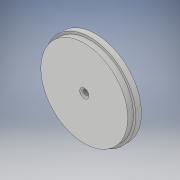
# Autodesk Inventor part: Cap
Saved by Autodesk Inventor 2019 (Build 230136000, 136)
## iProperties
Created: 2021-01-17
Part Number: Cap
Material: Типовые
Document SubType Name: Modeling
Designer: Dazer
Density: 1 g/cm^3
Appearance: По умолчанию
Author: Dazer
## iProperties of the stored document Cap_3DПЕЧАТЬ.ipt
Created: 2021-01-18
Part Number: Cap_3DПЕЧАТЬ
Material: Типовые
Document SubType Name: Modeling
Designer: Dazer
Density: 1 g/cm^3
Appearance: По умолчанию
Author: Dazer
Autodesk Inventor part; units mm, degrees
ref_plane "YZ Plane" through (0, 0, 0) normal (1, 0, 0) x (0, 1, 0)
ref_plane "XZ Plane" through (0, 0, 0) normal (0, 1, 0) x (-1, 0, 0)
ref_plane "XY Plane" through (0, 0, 0) normal (0, 0, 1) x (1, 0, 0)
sketch "Эскиз1" plane through (0, 0, 0) normal (0, 0, 1) x (1, 0, 0)
  circle A0 centre (0, 44.0756) radius 40
  point P0 (0, 0)
  dimension "d0" = 80
  constraints: 1 centre point
  measures "d0" diameter of A0
extrude "Выдавливание1" add sketch "Эскиз1" along normal blind 5
sketch "Эскиз2" plane through (0, 44.0756, 0) normal (0, 0, -1) x (-1, 0, 0)
  line L0 (0, 4) -> (-3.4641, 2)
  line L1 (-3.4641, 2) -> (-3.4641, -2)
  line L2 (-3.4641, -2) -> (0, -4)
  line L3 (0, -4) -> (3.421, -2.0249)
  line L4 (3.421, -2.0249) -> (3.4641, 2)
  line L5 (3.4641, 2) -> (0, 4)
  point P0 (0, -44.0756)
  point P1 (0, 0)
  constraints: 12 end point, 2 parallel
extrude "Выдавливание2" cut sketch "Эскиз2" against normal blind 4
sketch "Эскиз3" plane through (0, 44.0756, 5) normal (0, 0, 1) x (1, 0, 0)
  circle A0 centre (0, 0) radius 40 projected
  circle A1 centre (0, 0) radius 38
  point P0 (0, -44.0756)
  dimension "d5" = 2
  constraints: 1 centre point
  measures "d5" radial gap between concentric circles of A0 A1
extrude "Выдавливание3" add sketch "Эскиз3" along normal blind 5 contours A1
sketch "Эскиз5" plane through (0, 44.0756, 10) normal (0, 0, 1) x (1, 0, 0)
  circle A0 centre (0, 0) radius 38 projected
  point P0 (0, -44.0756)
hole "Отверстие1" at (0, 44.0756, 10) direction (0, 0, -1) diameter 4.5 end through all countersink diameter 8 countersink angle 90
